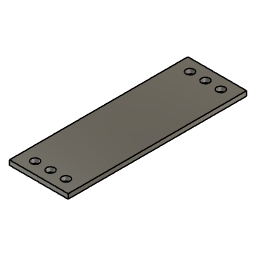
Suspension Axis Cover (Autodesk Fusion 360 design; units mm, degrees)
Autodesk Fusion 360 part; units mm, degrees
sketch "Sketch1" plane through (0, 0, 0) normal (0, 0, 1) x (1, 0, 0)
  line L0 (27, 38) -> (-27, 38)
  line L1 (-27, 38) -> (-27, -38)
  line L2 (-27, -38) -> (27, -38)
  line L3 (27, -38) -> (27, 38)
  line L4 (27, 38) -> (-27, -38) construction
  line L5 (-27, 38) -> (27, -38) construction
  line L6 (-27, 30) -> (27, 30)
  line L7 (0, 0) -> (5, 0)
  line L8 (0, 0) -> (0, 6)
  line L9 (-27, -30) -> (27, -30)
  line L10 (-12.5, 30) -> (-12.5, -30)
  line L11 (12.5, 30) -> (12.5, -30)
  line L12 (-12.5, 30) -> (-12.5, 38)
  line L13 (12.5, 30) -> (12.5, 38)
  circle A0 centre (0, 33) radius 1.7
  circle A1 centre (0, -33) radius 1.7
  line L14 (-12.5, -30) -> (-12.5, -38)
  line L15 (12.5, -30) -> (12.5, -38)
  circle A2 centre (-20.55, 33) radius 1.7
  circle A3 centre (-6.55, 33) radius 1.7
  circle A4 centre (20.55, 33) radius 1.7
  circle A5 centre (6.55, 33) radius 1.7
  circle A6 centre (-20.55, -33) radius 1.7
  circle A7 centre (-6.55, -33) radius 1.7
  circle A8 centre (6.55, -33) radius 1.7
  circle A9 centre (20.55, -33) radius 1.7
  dimension "d1" = 8
  dimension "d2" = 25
  dimension "d3" = 25
  dimension "d5" = 5
  dimension "d6" = 3.4
  dimension "d9" = 14
  dimension "d10" = 20.55
  dimension "d13" = 60
  dimension "d14" = 54
  constraint horizontal L0
  constraint perpendicular L0 L1
  constraint parallel L0 L2
  constraint parallel L1 L3
  constraint coincident L4 L7.start
  constraint coincident L5 L7.start
  constraint coincident L7.start L8.start
  constraint coincident L1 L6.start
  constraint coincident L3 L6.end
  constraint parallel L0 L6
  constraint parallel L0 L7
  constraint perpendicular L7 L8
  constraint symmetric L6.start L7 L9.start
  constraint symmetric L6.end L7 L9.end
  constraint coincident L6 L10.start
  constraint coincident L9 L10.end
  constraint perpendicular L9 L10
  constraint symmetric L8 L10.start L11.start
  constraint symmetric L8 L10.end L11.end
  constraint coincident L0 L12.end
  constraint perpendicular L6 L12
  constraint symmetric L8 L12.end L13.end
  constraint symmetric L7 A0 A1
  constraint symmetric L7 L10.start L10.end
  constraint symmetric L7 L12.end L14.end
  constraint symmetric L7 L11.start L11.end
  constraint symmetric L7 L13.end L15.end
  constraint equal A2 A3
  constraint equal A0 A3
  constraint symmetric L8 A2 A4
  constraint symmetric L8 A3 A5
  constraint symmetric L7 A2 A6
  constraint symmetric L7 A3 A7
  constraint symmetric L7 A4 A9
  constraint symmetric L7 A5 A8
  constraint collinear A0.centre A3.centre A5.centre
  constraint collinear A0.centre A2.centre A3.centre
  constraint collinear L7.start L8.end A0.centre
  measures "d1" distance of L0 L6
  measures "d2" distance of L10 L11
  measures "d3" distance of L12 L13
  measures "d5" distance of L0 A0.centre
  measures "d6" diameter of A0
  measures "d9" distance of A2.centre A3.centre
  measures "d10" distance of L8 A2.centre
  measures "d13" distance of L6 L9
  measures "d14" distance of L0.start L0.end
extrude "Extrude1" add sketch "Sketch1" along normal blind 2 contours L0 L6 L12 L13 | L6 L9 L10 L11 | L2 L9 L14 L15
equation "d10 = ( 41.1 / 2 ) * 1 mm"
